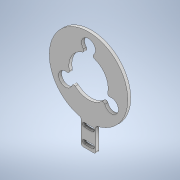
# Autodesk Inventor part: Деталь2_мозговорот
Saved by Autodesk Inventor 2021 (Build 250183000, 183)
## iProperties
Created: 2022-11-16
Part Number: Деталь2_мозговорот
Material: Типовые
Document SubType Name: Modeling
Designer: zmoze
Density: 1 g/cm^3
Appearance: По умолчанию
Author: zmoze
Autodesk Inventor part; units mm, degrees
ref_plane "YZ Plane" through (0, 0, 0) normal (1, 0, 0) x (0, 1, 0)
ref_plane "XZ Plane" through (0, 0, 0) normal (0, 1, 0) x (-1, 0, 0)
ref_plane "XY Plane" through (0, 0, 0) normal (0, 0, 1) x (1, 0, 0)
sketch "Эскиз1" plane through (0, 0, 0) normal (0, 0, 1) x (1, 0, 0)
  line L0 (17.5, 5) -> (-17.5, 5) construction
  line L1 (-17.5, 5) -> (-17.5, -5) construction
  line L2 (-17.5, -5) -> (17.5, -5) construction
  line L3 (17.5, -5) -> (17.5, 5) construction
  line L4 (17.5, 5) -> (-17.5, -5) construction
  line L5 (-17.5, 5) -> (17.5, -5) construction
  line L6 (12.8471, 5) -> (-11.1661, 5) construction
  circle A0 centre (0, 69.2906) radius 40
  circle A1 centre (0, 69.2906) radius 20
  line L7 (0, 69.2906) -> (0, 0) construction
  circle A2 centre (0, 96.3406) radius 7.05
  line L8 (-7.5, 5) -> (-7.5, 30)
  line L9 (7.5, 30) -> (7.5, 5)
  line L10 (-2, 49.2906) -> (2, 49.2906) construction
  line L11 (-7.5, 5) -> (7.5, 5)
  line L12 (-2, 90.7906) -> (2, 90.7906)
  line L13 (2, 90.7906) -> (2, 87.7906)
  line L14 (2, 87.7906) -> (-2, 87.7906)
  line L15 (-2, 87.7906) -> (-2, 90.7906)
  line L16 (-2, 90.7906) -> (2, 87.7906) construction
  line L17 (2, 90.7906) -> (-2, 87.7906) construction
  line L18 (-17.6195, 56.8085) -> (-19.6195, 60.2726)
  circle A3 centre (-23.426, 55.7656) radius 7.05
  line L19 (-17.0215, 61.7726) -> (-15.0215, 58.3085)
  line L20 (-19.6195, 60.2726) -> (-17.0215, 61.7726)
  line L21 (-15.0215, 58.3085) -> (-17.6195, 56.8085)
  line L22 (19.6195, 60.2726) -> (17.6195, 56.8085)
  circle A4 centre (23.426, 55.7656) radius 7.05
  line L23 (15.0215, 58.3085) -> (17.0215, 61.7726)
  line L24 (17.6195, 56.8085) -> (15.0215, 58.3085)
  line L25 (17.0215, 61.7726) -> (19.6195, 60.2726)
  point P0 (0, 89.2906)
  point P1 (0, 89.2906)
  point P2 (-17.3205, 59.2906)
  point P3 (17.3205, 59.2906)
  point P4 (18.2337, 61.0728)
  point P5 (18.5713, 60.8778)
  point P6 (16.5713, 57.4137)
  point P7 (16.2337, 57.6087)
  point P8 (-16.2337, 57.6087)
  point P9 (-16.5713, 57.4137)
  point P10 (-18.5713, 60.8778)
  point P11 (-18.2337, 61.0728)
  point P12 (-2, 89.1903)
  point P13 (-2, 89.5802)
  point P14 (2, 89.5802)
  point P15 (2, 89.1903)
  dimension "d3" = 40
  dimension "d4" = 14.1
  dimension "d0" = 80
  dimension "d9" = 35
  dimension "d10" = 25
  dimension "d11" = 10
  dimension "d12" = 15
  dimension "d14" = 7.5
  dimension "d30" = 4
  dimension "d31" = 3
  dimension "d34" = 360
  constraints: 52 end point, 4 midpoint, 4 parallel, 4 perpendicular, 4 point on line, 3 horizontal, 2 point on circle, 1 centre point, 1 coincident, 1 collinear, 1 vertical, 46 other
  measures "d0" diameter of A0
  measures "d9" distance of L1.end L2.end
  measures "d10" distance of L9.start L9.end
  measures "d11" distance of L2.end L0.start
  measures "d12" distance between parallel lines of L8 L9
  measures "d14" distance between parallel lines of L8 L7
  measures "d30" distance of L12.start L12.end
  measures "d31" distance of L14.end L12.start
extrude "Выдавливание1" add sketch "Эскиз1" along normal blind 3
fillet "Сопряжение1" radius 2 14 edges at (-7.5, 30, 1.5) (7.5, 30, 1.5) (-18.2337, 61.0728, 1.5) (-18.5713, 60.8778, 1.5) (-16.2337, 57.6087, 1.5) (-16.5713, 57.4137, 1.5) (-2, 89.1903, 1.5) (-2, 89.5802, 1.5) (2, 89.1903, 1.5) (2, 89.5802, 1.5) (18.5713, 60.8778, 1.5) (18.2337, 61.0728, 1.5) (16.5713, 57.4137, 1.5) (16.2337, 57.6087, 1.5)
sketch "Эскиз2" plane through (0, 0, 3) normal (0, 0, 1) x (1, 0, 0)
  circle A0 centre (0, 25) radius 2 construction
  circle A1 centre (0, 10) radius 2 construction
  line L0 (0, 0) -> (0, 43.9437)
  line L1 (0, 10) -> (0, 5)
  line L2 (-7.5, 5) -> (7.5, 5) projected
  arc A2 (19.5416, 65.0331) -> (6.0837, 88.3428) centre (0, 69.2906) ccw projected
  arc A3 (-4.1892, 25.1986) -> (4.1892, 25.1986) centre (0, 69.2906) ccw construction
  arc A4 (-4.3783, 23.2075) -> (4.3783, 23.2075) centre (0, 69.2906) ccw
  arc A5 (-4, 27.1896) -> (4, 27.1896) centre (0, 69.2906) ccw
  arc A6 (-4, 27.1896) -> (-4.3783, 23.2075) centre (-4.1892, 25.1986) ccw
  arc A7 (4.3783, 23.2075) -> (4, 27.1896) centre (4.1892, 25.1986) ccw
  arc A8 (-4.1396, 10.1447) -> (4.1396, 10.1447) centre (0, 69.2906) ccw construction
  arc A9 (-4.2793, 8.1496) -> (4.2793, 8.1496) centre (0, 69.2906) ccw
  arc A10 (-4, 12.1398) -> (4, 12.1398) centre (0, 69.2906) ccw
  arc A11 (-4, 12.1398) -> (-4.2793, 8.1496) centre (-4.1396, 10.1447) ccw
  arc A12 (4.2793, 8.1496) -> (4, 12.1398) centre (4.1396, 10.1447) ccw
  dimension "d24" = 15
  dimension "d25" = 5
  dimension "d26" = 4
  dimension "d27" = 4
  dimension "d39" = 4
  dimension "d40" = 8
  dimension "d41" = 4
  dimension "d42" = 8
  constraints: 22 point on circle, 12 centre point, 8 tangent, 4 end point, 2 coincident, 2 point on line, 1 midpoint, 1 vertical
  measures "d24" distance of A0.centre L1.start
  measures "d25" distance of L1.start L1.end
  measures "d26" diameter of A1
  measures "d27" diameter of A0
  measures "d39" radial gap between concentric circles of A4 A5
  measures "d40" distance of A5.start A5.end
  measures "d41" radial gap between concentric circles of A9 A10
  measures "d42" distance of A10.end A10.start
extrude "Выдавливание2" cut sketch "Эскиз2" against normal blind 4
fillet "Сопряжение2" radius 2 2 edges at (7.5, 5, 1.5) (-7.5, 5, 1.5)
